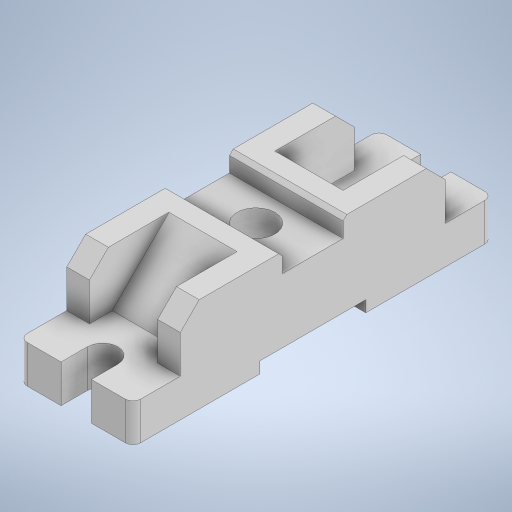
# Autodesk Inventor part: esercizio 040.30 03-02-2023
Saved by Autodesk Inventor 2023 (Build 270158000, 158)
## iProperties
Created: 2023-03-02
Part Number: esercizio 040.30 03-02-2023
Material: Generico
Document SubType Name: Modeling
Designer: Admin
Density: 1 g/cm^3
Appearance: Default
Author: Admin
Autodesk Inventor part; units mm, degrees
ref_plane "YZ Plane" through (0, 0, 0) normal (1, 0, 0) x (0, 1, 0)
ref_plane "XZ Plane" through (0, 0, 0) normal (0, 1, 0) x (-1, 0, 0)
ref_plane "XY Plane" through (0, 0, 0) normal (0, 0, 1) x (1, 0, 0)
sketch "Schizzo1" plane through (0, 0, 0) normal (0, 1, 0) x (-1, 0, 0)
  line L0 (0, 0) -> (15, 0) construction
  line L1 (15, 0) -> (15, -47.5)
  line L2 (15, -47.5) -> (4, -47.5)
  line L3 (4, -47.5) -> (4, -40.5)
  line L4 (0, 0) -> (0, -36.5) construction
  arc A0 (4, -40.5) -> (0, -36.5) centre (0, -40.5) ccw
  arc A1 (0, -5) -> (5, 0) centre (0, 0) ccw
  line L5 (0, 0) -> (0, -8) construction
  line L6 (0, -8) -> (15, -8)
  line L7 (15, 0) -> (15, -14)
  line L8 (15, -14) -> (0, -14)
  line L9 (15, -35) -> (9, -35)
  line L10 (9, -35) -> (9, -14)
  line L11 (0, 0) -> (-15, 0) construction
  line L12 (-15, 0) -> (-15, -47.5)
  line L13 (-15, -47.5) -> (-4, -47.5)
  line L14 (-4, -47.5) -> (-4, -40.5)
  arc A2 (0, -36.5) -> (-4, -40.5) centre (0, -40.5) ccw
  arc A3 (-5, 0) -> (0, -5) centre (0, 0) ccw
  line L15 (0, -8) -> (-15, -8)
  line L16 (-15, 0) -> (-15, -14)
  line L17 (-15, -14) -> (0, -14)
  line L18 (-15, -35) -> (-9, -35)
  line L19 (-9, -35) -> (-9, -14)
  line L20 (15, 0) -> (15, 47.5)
  line L21 (15, 47.5) -> (4, 47.5)
  line L22 (4, 47.5) -> (4, 40.5)
  line L23 (0, 0) -> (0, 36.5) construction
  arc A4 (0, 36.5) -> (4, 40.5) centre (0, 40.5) ccw
  arc A5 (5, 0) -> (0, 5) centre (0, 0) ccw
  line L24 (0, 0) -> (0, 8) construction
  line L25 (0, 8) -> (15, 8)
  line L26 (15, 0) -> (15, 14)
  line L27 (15, 14) -> (0, 14)
  line L28 (15, 35) -> (9, 35)
  line L29 (9, 35) -> (9, 14)
  arc A6 (-4, 40.5) -> (0, 36.5) centre (0, 40.5) ccw
  line L30 (-15, 47.5) -> (-4, 47.5)
  line L31 (-4, 47.5) -> (-4, 40.5)
  line L32 (-15, 35) -> (-9, 35)
  line L33 (-15, 14) -> (0, 14)
  line L34 (-9, 35) -> (-9, 14)
  line L35 (-15, 0) -> (-15, 47.5)
  line L36 (0, 8) -> (-15, 8)
  arc A7 (0, 5) -> (-5, 0) centre (0, 0) ccw
  line L37 (-15, 0) -> (-15, 14)
  dimension "d0" = 15
  dimension "d1" = 47.5
  dimension "d2" = 11
  dimension "d5" = 5
  dimension "d6" = 8
  dimension "d7" = 14
  dimension "d8" = 6
  constraints: 76 end point, 31 symmetric about line, 26 point on line, 16 point on circle, 8 centre point, 5 perpendicular, 4 coincident, 2 vertical, 1 horizontal, 1 parallel, 1 tangent, 6 other
  measures "d0" distance of L0.start L0.end
  measures "d1" distance of L0.end L1.end
  measures "d2" distance of L1.end L2.end
  measures "d5" radius of A1
  measures "d6" distance of L5.start L5.end
  measures "d7" distance of L0.end L7.end
  measures "d8" distance of L9.start L9.end
extrude "Estrusione1" add sketch "Schizzo1" along normal blind 10 contours L1 L2 L3 A0 A2 L14 L13 L12 L18 L19 L17 L8 L10 L9 | L28 L29 L27 L33 L34 L32 L35 L30 L31 A6 A4 L22 L21 L20
extrude "Estrusione2" add sketch "Schizzo1" along normal blind 25 contours L1 L8 L17 L12 L15 L6 | L25 L36 L35 L33 L27 L20 | L1 L9 L10 L8 | L27 L29 L28 L20 | L17 L19 L18 L12 | L35 L32 L34 L33
extrude "Estrusione3" add sketch "Schizzo1" along normal blind 20 contours L1 L6 L15 L12 L35 L36 L25 L20
sketch "Schizzo1 outline for Estrusione4" plane through (0, 0, 0) normal (0, 1, 0) x (-1, 0, 0)
  line L0 (-15, 0) -> (-15, -14)
  line L1 (-15, 14) -> (-15, 0)
  line L2 (-15, -14) -> (0, -14)
  line L3 (0, 14) -> (-15, 14)
  line L4 (0, -14) -> (15, -14)
  line L5 (15, 14) -> (0, 14)
  line L6 (15, -14) -> (15, 0)
  line L7 (15, 0) -> (15, 14)
  arc A0 (0, -5) -> (-5, 0) centre (0, 0) cw
  arc A1 (5, 0) -> (0, -5) centre (0, 0) cw
  arc A2 (0, 5) -> (5, 0) centre (0, 0) cw
  arc A3 (-5, 0) -> (0, 5) centre (0, 0) cw
extrude "Estrusione4" cut sketch "Schizzo1 outline for Estrusione4" along normal blind 3
chamfer "Smusso1" distance 15 angle 45 1 edges at (0, 10, 14) measured on face at (-3, 15, 14)
chamfer "Smusso2" distance 15 angle 45 1 edges at (0, 10, -14) measured on face at (3, 15, -14)
chamfer "Smusso3" distance 5 angle 45 2 edges at (-12, 25, -35) (12, 25, -35) measured on face at (3, 25, -10)
chamfer "Smusso4" distance 5 angle 45 2 edges at (12, 25, 35) (-12, 25, 35) measured on face at (-3, 25, 10)
fillet "Raccordo1" radius 2 4 edges at (-15, 5, -47.5) (-15, 5, 47.5) (15, 5, 47.5) (15, 5, -47.5)
chamfer "Smusso5" distance 1 angle 45 1 edges at (0, 25, -8) measured on face at (-3, 25, -10)
chamfer "Smusso6" distance 1 angle 45 1 edges at (0, 25, 8) measured on face at (-3, 25, 10)
